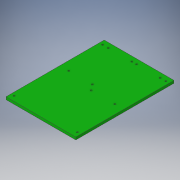
# Autodesk Inventor part: ModBoard-Bottom
Saved by Autodesk Inventor 2018 (Build 220112000, 112)
## iProperties
Created: 2017-12-22
Part Number: ModBoard-Bottom
Material: Generic
Document SubType Name: Modeling
Designer: jklei
Density: 1 g/cm^3
Appearance: Default
Author: jklei
Autodesk Inventor part; units mm, degrees
ref_plane "YZ Plane" through (0, 0, 0) normal (1, 0, 0) x (0, 1, 0)
ref_plane "XZ Plane" through (0, 0, 0) normal (0, 1, 0) x (-1, 0, 0)
ref_plane "XY Plane" through (0, 0, 0) normal (0, 0, 1) x (1, 0, 0)
sketch "Sketch1" plane through (0, 0, 0) normal (0, 1, 0) x (-1, 0, 0)
  line L0 (0, 0) -> (-171.45, 0)
  line L1 (-171.45, 0) -> (-171.45, -241.3)
  line L2 (-171.45, -241.3) -> (0, -241.3)
  line L3 (0, -241.3) -> (0, 0)
  dimension "d0" = 171.45
  dimension "d1" = 241.3
  constraints: 8 end point, 2 parallel, 1 horizontal, 1 perpendicular
  measures "d0" distance of L2.end L1.end
  measures "d1" distance of L1.end L0.end
extrude "Extrusion1" add sketch "Sketch1" along normal blind 6.35
sketch "Sketch2" plane through (0, 6.35, 0) normal (0, 1, 0) x (1, 0, 0)
  line L0 (0, 0) -> (8, 0)
  line L1 (0, 0) -> (171.45, 0) projected
  line L2 (8, 0) -> (8, 12)
  line L3 (171.45, 0) -> (163.45, 0)
  line L4 (163.45, 0) -> (163.45, 12)
  line L5 (171.45, 241.3) -> (0, 241.3) projected
  line L6 (0, 241.3) -> (8, 241.3)
  line L7 (8, 241.3) -> (8, 229.3)
  line L8 (171.45, 241.3) -> (163.45, 241.3)
  line L9 (163.45, 241.3) -> (163.45, 229.3)
  circle A0 centre (8, 229.3) radius 2.1
  circle A1 centre (163.45, 229.3) radius 2.1
  circle A2 centre (163.45, 12) radius 2.1
  circle A3 centre (8, 12) radius 2.1
  dimension "d4" = 8
  dimension "d5" = 12
  dimension "d6" = 8
  dimension "d7" = 12
  dimension "d8" = 8
  dimension "d9" = 12
  dimension "d10" = 8
  dimension "d11" = 12
  dimension "d12" = 4.2
  dimension "d13" = 4.2
  dimension "d14" = 4.2
  dimension "d15" = 4.2
  constraints: 16 end point, 4 centre point, 4 coincident, 4 perpendicular, 4 point on line
  measures "d4" distance of L0.start L0.end
  measures "d5" distance of L0.end L2.end
  measures "d6" distance of L1.end L3.end
  measures "d7" distance of L3.end L4.end
  measures "d8" distance of L5.end L6.end
  measures "d9" distance of L6.end L7.end
  measures "d10" distance of L5.start L8.end
  measures "d11" distance of L8.end L9.end
  measures "d12" diameter of A0
  measures "d13" diameter of A1
  measures "d14" diameter of A2
  measures "d15" diameter of A3
extrude "Extrusion2" cut sketch "Sketch2" against normal blind 25.4
sketch "Sketch3" plane through (0, 6.35, 0) normal (0, 1, 0) x (1, 0, 0)
  circle A0 centre (163.45, 12) radius 2.1 projected
  circle A1 centre (8, 229.3) radius 2.1 projected
  circle A2 centre (163.45, 229.3) radius 2.1 projected
  circle A3 centre (8, 12) radius 2.1 projected
  line L0 (0, 0) -> (171.45, 0) projected
  line L1 (171.45, 0) -> (171.45, 241.3) projected
  line L2 (171.45, 241.3) -> (0, 241.3) projected
  line L3 (0, 241.3) -> (0, 0) projected
  line L4 (8, 229.3) -> (22, 229.3)
  circle A4 centre (22, 229.3) radius 2.1
  line L5 (22, 229.3) -> (80, 229.3)
  circle A5 centre (80, 229.3) radius 2.1
  line L6 (163.45, 229.3) -> (149.45, 229.3)
  line L7 (149.45, 229.3) -> (91.45, 229.3)
  circle A6 centre (149.45, 229.3) radius 2.1
  circle A7 centre (91.45, 229.3) radius 2.1
  circle A8 centre (149.45, 118.048) radius 2.1
  circle A9 centre (91.45, 118.048) radius 2.1
  line L8 (80, 229.3) -> (80, 132.2974)
  circle A10 centre (80, 132.2974) radius 2.1
  circle A11 centre (22, 132.2974) radius 2.1
  dimension "d18" = 14
  dimension "d19" = 4.2
  dimension "d20" = 58
  dimension "d21" = 4.2
  dimension "d22" = 14
  dimension "d23" = 58
  dimension "d24" = 4.2
  dimension "d25" = 4.2
  dimension "d28" = 4.2
  dimension "d29" = 111.252
  dimension "d30" = 0
  dimension "d31" = 4.2
  dimension "d32" = 58
  dimension "d33" = 111.252
  dimension "d34" = 97.0026
  dimension "d35" = 4.2
  dimension "d36" = 4.2
  dimension "d37" = 0
  dimension "d38" = 97.0026
  constraints: 10 end point, 8 centre point, 5 coincident, 3 horizontal, 1 point on line, 1 vertical
  measures "d18" distance of L4.start L4.end
  measures "d19" diameter of A4
  measures "d20" distance of L5.start L5.end
  measures "d21" diameter of A5
  measures "d22" distance of L6.start L6.end
  measures "d23" distance of L6.end L7.end
  measures "d24" diameter of A6
  measures "d25" diameter of A7
  measures "d28" diameter of A8
  measures "d29" distance of A8.centre L6.end
  measures "d30" horizontal distance of A6.centre A8.centre
  measures "d31" diameter of A9
  measures "d32" distance of A8.centre A9.centre
  measures "d33" distance of A7.centre A9.centre
  measures "d34" distance of L8.start L8.end
  measures "d35" diameter of A10
  measures "d36" diameter of A11
  measures "d37" vertical distance of L8.end A11.centre
  measures "d38" distance of L4.end A11.centre
extrude "Extrusion3" cut sketch "Sketch3" against normal blind 25.4 contours A4 L5 L4 | L4 L5 A4 | A5 L8 L5 | L5 L8 A5 | A6 L7 L6 | L6 L7 A6 | A7 | A8 | A9 | A10 | A11
body "Solid1"
